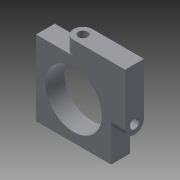
# Autodesk Inventor part: HW 5 Part 5
Saved by Autodesk Inventor 2015 (Build 190159000, 159)
## iProperties
Created: 2016-02-07
Part Number: HW 5 Part 5
Material: Generic
Document SubType Name: Modeling
Designer: Melissa
Density: 1 g/cm^3
Appearance: Default
Author: Melissa
Autodesk Inventor part; units mm, degrees
ref_plane "YZ Plane" through (0, 0, 0) normal (1, 0, 0) x (0, 1, 0)
ref_plane "XZ Plane" through (0, 0, 0) normal (0, 1, 0) x (-1, 0, 0)
ref_plane "XY Plane" through (0, 0, 0) normal (0, 0, 1) x (1, 0, 0)
sketch "Sketch1" plane through (0, 0, 0) normal (0, 0, 1) x (1, 0, 0)
  line L0 (0, 0) -> (101.6, 0)
  line L1 (101.6, 0) -> (101.6, 50.8)
  line L2 (50.8, 101.6) -> (0, 101.6)
  line L3 (0, 101.6) -> (0, 0)
  circle A0 centre (50.8, 50.8) radius 38.1
  line L4 (50.8, 101.6) -> (50.8, 120.65)
  line L5 (50.8, 120.65) -> (120.65, 120.65)
  line L6 (101.6, 50.8) -> (120.65, 50.8)
  line L7 (120.65, 50.8) -> (120.65, 120.65)
  dimension "d0" = 101.6
  dimension "d1" = 101.6
  dimension "d6" = 76.2
  dimension "d7" = 50.8
  dimension "d8" = 50.8
  dimension "d9" = 19.05
  dimension "d10" = 19.05
  constraints: 16 end point, 5 perpendicular, 2 horizontal, 1 centre point
  measures "d0" distance of L2.end L0.start
  measures "d1" distance of L0.start L0.end
  measures "d6" diameter of A0
  measures "d7" distance from line of L0 A0.centre
  measures "d8" distance from line of L3 A0.centre
  measures "d9" distance of L2.start L4.end
  measures "d10" distance of L1.end L6.end
extrude "Extrusion1" add sketch "Sketch1" along normal blind 25.4
sketch "Sketch2" plane through (0, 101.6, 0) normal (0, 1, 0) x (1, 0, 0)
  line L0 (50.8, 0) -> (0, 0) projected
  circle A0 centre (50.8, -12.7) radius 12.7
  line L1 (50.8, -25.4) -> (0, -25.4) projected
  line L2 (50.8, 0) -> (50.8, -25.4) projected
  dimension "d16" = 25.4
  dimension "d17" = 0
  constraints: 1 centre point, 1 tangent
  measures "d16" diameter of A0
  measures "d17" distance from line of L2 A0.centre
extrude "Extrusion2" add sketch "Sketch2" along normal blind 19.05
sketch "Sketch3" plane through (120.65, 120.65, 25.4) normal (0, 1, 0) x (1, 0, 0)
  arc A0 (-69.85, 25.4) -> (-69.85, 0) centre (-69.85, 12.7) ccw projected
  circle A1 centre (-69.85, 12.7) radius 6.35
  point P0 (-120.65, 25.4)
  dimension "d21" = 12.7
  constraints: 1 centre point, 1 coincident
  measures "d21" diameter of A1
extrude "Extrusion3" cut sketch "Sketch3" against normal blind 19.05
sketch "Sketch4" plane through (120.65, 50.8, 0) normal (1, 0, 0) x (0, 0, -1)
  circle A0 centre (-12.7, 0) radius 12.7
  line L0 (0, -50.8) -> (0, 0) projected
  line L1 (0, 0) -> (-25.4, 0) projected
  dimension "d24" = 25.4
  dimension "d25" = 0
  constraints: 1 centre point, 1 tangent
  measures "d24" diameter of A0
  measures "d25" distance from line of L1 A0.centre
extrude "Extrusion4" add sketch "Sketch4" against normal blind 19.05
sketch "Sketch5" plane through (120.65, 120.65, 25.4) normal (1, 0, 0) x (0, 0, -1)
  arc A0 (0, -69.85) -> (25.4, -69.85) centre (12.7, -69.85) ccw projected
  circle A1 centre (12.7, -69.85) radius 6.35
  point P0 (25.4, -120.65)
  dimension "d28" = 12.7
  constraints: 1 centre point, 1 coincident
  measures "d28" diameter of A1
extrude "Extrusion5" cut sketch "Sketch5" against normal blind 19.05
equation "\"d1\" = d0"
equation "\"d6\" = 0.75 * d0"
equation "\"d7\" = d8"
equation "\"d8\" = 0.5 * d0"
equation "\"d21\" = 0.5 * d16"
equation "\"d24\" = d16"
equation "\"d28\" = d21"
body "Solid1"
